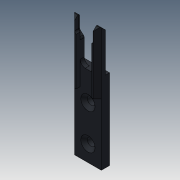
# Autodesk Inventor part: J007803
Saved by Autodesk Inventor 2018.3 (Build 223284000, 284)
## iProperties
Created: 2018-04-30
Material: VERO BLACK
Vendor: HHMI: JRC - ID&F
Document SubType Name: Modeling
Designer: arnoldj
Density: 1.17 g/cm^3
Appearance: Black Anodize
Part Number: J007803
Description: NEUROPIXEL 3A PROBE BASE
Project: COMMON
RuleStatus: InUse
AfterDocSave0: file://Part Number Cleaner
LAB/DEPT: COMMON
REQUESTING SCIENTIST: COMMON
SURFACE ROUGHNESS: 63 Ra
DESIGN DEPARTMENT: HHMI: JRC - ID&F
SPECIAL FINISH: NONE
ALTERED ITEM PART NUMBER: N/A
ALTERED ITEM VENDOR: N/A
ALTERED ITEM DESCRIPTION: N/A
Author: arnoldj
Revision Number: 0
Autodesk Inventor part; units mm, degrees
ref_plane "YZ Plane" through (0, 0, 0) normal (1, 0, 0) x (0, 1, 0)
ref_plane "XZ Plane" through (0, 0, 0) normal (0, 1, 0) x (-1, 0, 0)
ref_plane "XY Plane" through (0, 0, 0) normal (0, 0, 1) x (1, 0, 0)
sketch "Sketch1" plane through (0, 0, 0) normal (0, 0, 1) x (1, 0, 0)
  line L0 (0, 26.67) -> (0, -26.67) projected
  line L1 (-5.7785, 0) -> (5.7785, 0) projected
  line L2 (4.1275, -19.05) -> (-4.1275, -19.05)
  line L3 (-4.1275, -19.05) -> (-4.1275, 19.05)
  line L4 (-4.1275, 19.05) -> (4.1275, 19.05)
  line L5 (4.1275, 19.05) -> (4.1275, -19.05)
  line L6 (4.1275, -19.05) -> (-4.1275, 19.05) construction
  line L7 (-4.1275, -19.05) -> (4.1275, 19.05) construction
  point P0 (0, 0)
  point P1 (0, -14.05)
  point P2 (0, -3.05)
  dimension "d0" = 38.1
  dimension "d1" = 8.255
  dimension "d2" = 5
  dimension "d3" = 11
  constraints: 12 end point, 2 midpoint, 2 parallel, 2 point on line, 1 horizontal, 1 perpendicular
  measures "d0" distance of L2.end L3.end
  measures "d1" distance of L3.end L4.end
  measures "d2" distance from line of point (0, -14.05) L2
  measures "d3" distance of point (0, -14.05) point (0, -3.05)
extrude "Extrusion1" add sketch "Sketch1" along normal blind 3.81
sketch "Sketch5" plane through (0, 0, 3.81) normal (0, 0, 1) x (1, 0, 0)
  point P0 (0, 0)
  point P1 (0, -3.05)
  point P2 (0, -14.05)
hole "Hole2" at (0, -3.05, 3.81) at (0, -14.05, 3.81) direction (0, 0, -1) diameter 1.27 end through all
sketch "Sketch2" plane through (0, 0, 0) normal (0, 0, -1) x (-1, 0, 0)
  line L0 (4.1275, 19.05) -> (-4.1275, 19.05) projected
  line L1 (-3.8354, 19.05) -> (-3.8354, 14.0205)
  line L2 (-3.8354, 14.0205) -> (-2.413, 12.827)
  line L3 (-2.413, 12.827) -> (2.413, 12.827)
  line L4 (2.413, 12.827) -> (3.8354, 14.0205)
  line L5 (3.8354, 14.0205) -> (3.8354, 19.05)
  line L6 (0, -26.67) -> (0, 26.67) projected
  line L7 (-6.6675, 0) -> (6.6675, 0) projected
  point P0 (0, 0)
  dimension "d13" = 7.6708
  dimension "d14" = 6.223
  dimension "d15" = 4.826
  dimension "d16" = 3.8354
  dimension "d17" = 2.413
  dimension "d18" = 140
  constraints: 10 end point, 2 point on line, 1 equal length, 1 parallel, 1 perpendicular, 1 vertical
  measures "d13" distance between parallel lines of L5 L1
  measures "d14" distance between parallel lines of L0 L3
  measures "d15" distance of L2.end L3.end
  measures "d16" distance between parallel lines of L5 L6
  measures "d17" distance from line of L6 L3.end
  measures "d18" angle of L4 L3
extrude "Extrusion2" cut sketch "Sketch2" against normal blind 2.54
sketch "Sketch3" plane through (0, 0, 0) normal (0, 0, -1) x (-1, 0, 0)
  line L0 (-3.8354, 19.05) -> (3.8354, 19.05) projected
  line L1 (-3.8354, 14.0205) -> (-3.8354, 19.05) projected
  line L2 (-2.413, 12.827) -> (-3.8354, 14.0205) projected
  line L3 (2.413, 12.827) -> (-2.413, 12.827) projected
  line L4 (3.8354, 14.0205) -> (2.413, 12.827) projected
  line L5 (3.8354, 19.05) -> (3.8354, 14.0205) projected
  line L6 (0, -26.67) -> (0, 26.67) projected
  line L7 (2.8575, 14.605) -> (-2.8575, 14.605)
  line L8 (-2.8575, 14.605) -> (-2.8575, 19.05)
  line L9 (-2.8575, 19.05) -> (2.8575, 19.05)
  line L10 (2.8575, 19.05) -> (2.8575, 14.605)
  line L11 (2.8575, 14.605) -> (-2.8575, 19.05) construction
  line L12 (-2.8575, 14.605) -> (2.8575, 19.05) construction
  line L13 (2.413, 5.715) -> (-2.413, 5.715)
  line L14 (-2.413, 5.715) -> (-2.413, 14.605)
  line L15 (-2.413, 14.605) -> (2.413, 14.605)
  line L16 (2.413, 14.605) -> (2.413, 5.715)
  line L17 (2.413, 5.715) -> (-2.413, 14.605) construction
  line L18 (-2.413, 5.715) -> (2.413, 14.605) construction
  point P0 (0, 0)
  point P1 (0, 16.8275)
  point P2 (0, 10.16)
  dimension "d21" = 5.715
  dimension "d22" = 4.826
  dimension "d23" = 8.89
  dimension "d24" = 4.445
  constraints: 24 end point, 4 midpoint, 4 parallel, 4 point on line, 2 horizontal, 2 perpendicular
  measures "d21" distance of L7.start L7.end
  measures "d22" distance of L13.start L13.end
  measures "d23" distance of L13.end L14.end
  measures "d24" distance of L7.end L8.end
extrude "Extrusion3" cut sketch "Sketch3" against normal through all contours L0 L6 L7 L8 | L0 L10 L7 L6 | L14 L7 L6 L3 | L3 L6 L13 L14 | L7 L16 L3 L6 | L3 L16 L13 L6
fillet "Fillet1" radius 0.7937 4 edges at (3.8354, 14.0205, 1.27) (2.413, 12.827, 1.27) (-2.413, 12.827, 1.27) (-3.8354, 14.0205, 1.27)
fillet "Fillet2" radius 0.7937 2 edges at (-2.8575, 14.605, 3.175) (2.8575, 14.605, 3.175)
sketch "Sketch6" plane through (0, 0, 0) normal (0, 0, -1) x (-1, 0, 0)
  line L0 (0, -26.67) -> (0, 26.67) projected
  line L1 (-8.89, 0) -> (8.89, 0) projected
  line L2 (6.35, 5.715) -> (-6.35, 5.715)
  line L3 (-6.35, 5.715) -> (-6.35, 19.05)
  line L4 (-6.35, 19.05) -> (6.35, 19.05)
  line L5 (6.35, 19.05) -> (6.35, 5.715)
  line L6 (6.35, 5.715) -> (-6.35, 19.05) construction
  line L7 (-6.35, 5.715) -> (6.35, 19.05) construction
  line L8 (-3.8354, 19.05) -> (-4.1275, 19.05) projected
  point P0 (0, 0)
  point P1 (0, 12.3825)
  dimension "d50" = 12.7
  dimension "d51" = 5.715
  dimension "d52" = 0
  constraints: 12 end point, 2 midpoint, 2 parallel, 1 horizontal, 1 perpendicular, 1 point on line
  measures "d50" distance of L3.end L4.end
  measures "d51" distance between parallel lines of L1 L2
  measures "d52" distance between parallel lines of L4 L8
extrude "Extrusion5" cut sketch "Sketch6" against normal blind 1.27
chamfer "Chamfer1" distance 1.27 angle 45 2 edges at (3.9815, 19.05, 1.27) (-3.9814, 19.05, 1.27)
chamfer "Chamfer2" distance 1.016 angle 45 2 edges at (3.4925, 19.05, 3.81) (-3.4925, 19.05, 3.81)
sketch "Sketch7" plane through (0, 0, 3.81) normal (0, 0, 1) x (1, 0, 0)
  line L0 (-4.1275, 18.034) -> (-2.8575, 18.034) projected
  line L1 (-4.1275, 18.034) -> (-4.1275, -19.05) projected
  line L2 (-4.1275, -19.05) -> (4.1275, -19.05) projected
  line L3 (4.1275, -19.05) -> (4.1275, 18.034) projected
  line L4 (2.8575, 18.034) -> (4.1275, 18.034) projected
  line L5 (2.8575, 18.034) -> (2.8575, 15.3178) projected
  arc A0 (2.413, 14.605) -> (2.8575, 15.3178) centre (2.0638, 15.3178) ccw projected
  line L6 (2.413, 14.605) -> (2.413, 5.715) projected
  line L7 (2.413, 5.715) -> (-2.413, 5.715) projected
  line L8 (-2.413, 5.715) -> (-2.413, 14.605) projected
  arc A1 (-2.8575, 15.3178) -> (-2.413, 14.605) centre (-2.0637, 15.3178) ccw projected
  line L9 (-2.8575, 15.3178) -> (-2.8575, 18.034) projected
  circle A2 centre (0, -3.05) radius 0.635 projected
  circle A3 centre (0, -14.05) radius 0.635 projected
  line L10 (-4.1275, -19.05) -> (4.1275, -19.05)
  line L11 (4.1275, -19.05) -> (4.1275, 0)
  line L12 (4.1275, 0) -> (-4.1275, 0)
  line L13 (-4.1275, 0) -> (-4.1275, -19.05)
  line L14 (-6.6675, 0) -> (6.6675, 0) projected
  line L15 (0, 26.67) -> (0, -26.67) projected
  line L16 (2.413, 0) -> (-2.413, 0)
  line L17 (-2.413, 0) -> (-2.413, 5.715)
  line L18 (-2.413, 5.715) -> (2.413, 5.715)
  line L19 (2.413, 5.715) -> (2.413, 0)
  line L20 (2.413, 0) -> (-2.413, 5.715) construction
  line L21 (-2.413, 0) -> (2.413, 5.715) construction
  point P0 (0, 0)
  point P1 (0, 2.8575)
  dimension "d55" = 0
  dimension "d58" = 0
  constraints: 20 end point, 4 parallel, 2 horizontal, 2 midpoint, 2 perpendicular, 2 point on line
  measures "d55" distance between parallel lines of L14 L12
  measures "d58" distance between parallel lines of L12 L16
extrude "Extrusion6" cut sketch "Sketch7" against normal blind 1.27 contours L12 L15 A2 A3 L2 L1 | L15 A3 A2 L12 L3 L2
hole "Hole3" at (0, -3.05, 2.54) direction (0, 0, -1) diameter 2.3876 end through all countersink diameter 4.3942 countersink angle 90 clearance for "Flat Head Machine Screw" size "M2" standard "Ansi Metric M Profile"
hole "Hole4" at (0, -14.05, 2.54) direction (0, 0, -1) diameter 2.3876 end through all countersink diameter 4.3942 countersink angle 90 clearance for "Flat Head Machine Screw" size "M2" standard "Ansi Metric M Profile"
extrude "Extrusion7" cut sketch "Sketch7" against normal up to surface (1.27 mm away) contours L17 L7 L15 L12 | L15 L7 L19 L12
fillet "Fillet3" radius 1.5875 2 edges at (2.413, 5.715, 1.905) (-2.413, 5.715, 1.905)
chamfer "Chamfer4" distance 1.27 angle 45 2 edges at (-4.1275, 9.017, 3.81) (4.1275, 9.017, 3.81)
equation "\"d16\" = 0.5 * d13"
equation "\"d17\" = 0.5 * d15"
body "Solid1"
